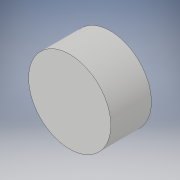
# Autodesk Inventor part: AC_Cylinder_9DecRadius
Saved by Autodesk Inventor 2017 (Build 210142000, 142)
## iProperties
Created: 2016-11-01
Part Number: AC_Cylinder_9DecRadius
Material: Generic
Document SubType Name: Modeling
Designer: aj
Density: 1 g/cm^3
Appearance: Default
Author: aj
Autodesk Inventor part; units mm, degrees
ref_plane "YZ Plane" through (0, 0, 0) normal (1, 0, 0) x (0, 1, 0)
ref_plane "XZ Plane" through (0, 0, 0) normal (0, 1, 0) x (-1, 0, 0)
ref_plane "XY Plane" through (0, 0, 0) normal (0, 0, 1) x (1, 0, 0)
sketch "Sketch1" plane through (0, 0, 0) normal (0, 0, 1) x (1, 0, 0)
  circle A0 centre (0, 0) radius 10.1235
  dimension "d0" = 10.1235
  constraints: 1 centre point, 1 coincident
  measures "d0" radius of A0
extrude "Extrusion1" add sketch "Sketch1" along normal blind 10
body "Solid1"
